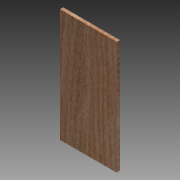
# Autodesk Inventor part: bottom2 battery holder
Saved by Autodesk Inventor 2014 (Build 180170000, 170)
## iProperties
Created: 2016-02-01
Part Number: bottom2 battery holder
Material: Generic
Document SubType Name: Modeling
Designer: sametj
Density: 1 g/cm^3
Appearance: Default
Author: sametj
Autodesk Inventor part; units mm, degrees
ref_plane "YZ Plane" through (0, 0, 0) normal (1, 0, 0) x (0, 1, 0)
ref_plane "XZ Plane" through (0, 0, 0) normal (0, 1, 0) x (-1, 0, 0)
ref_plane "XY Plane" through (0, 0, 0) normal (0, 0, 1) x (1, 0, 0)
sketch "Sketch1" plane through (0, 0, 0) normal (0, 0, 1) x (1, 0, 0)
  line L0 (37.0694, -105.5511) -> (-77.2306, -105.5511)
  line L1 (-77.2306, -105.5511) -> (-77.2306, 123.0489)
  line L2 (-77.2306, 123.0489) -> (37.0694, 123.0489)
  line L3 (37.0694, 123.0489) -> (37.0694, -105.5511)
  line L4 (37.0694, -105.5511) -> (-77.2306, 123.0489) construction
  line L5 (-77.2306, -105.5511) -> (37.0694, 123.0489) construction
  point P0 (0, 0)
  point P1 (-20.0806, 8.7489)
  dimension "d0" = 114.3
  dimension "d1" = 228.6
  constraints: 12 end point, 2 midpoint, 2 parallel, 1 horizontal, 1 perpendicular
  measures "d0" distance of L1.end L2.end
  measures "d1" distance of L0.end L1.end
extrude "Extrusion1" add sketch "Sketch1" along normal blind 6.35
body "Solid1"
